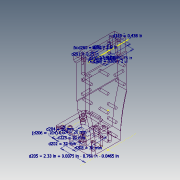
# Autodesk Inventor part: J003055
Saved by Autodesk Inventor 2015 SP1 (Build 190203100, 203)
## iProperties
Created: 2014-12-15
Material: ALUMINUM, 6061-T651
Vendor: HHMI: JFRC - ID&F
Document SubType Name: Modeling
Designer: ARNOLDJ
Density: 2.7 g/cm^3
Mass: 360.292 g
Surface Area: 312.552 cm^2
Volume: 133.442 cm^3
Part Number: J003055
Description: MBS OUTER POSARM
Appearance: Polished Brushed
Project: P-201804
RuleStatus: InUse
AfterDocSave0: file://Part Number Cleaner
LAB/DEPT: SVOBODA (LAB)
REQUESTING SCIENTIST: SOFRONIEW, NICK
SURFACE ROUGHNESS: 63 Ra
DESIGN DEPARTMENT: HHMI: JRC - ID&F
SPECIAL FINISH: ANODIZE PER MIL-A-8625F, TYPE II, CLASS 2 (BLACK)
ALTERED ITEM PART NUMBER: N/A
ALTERED ITEM VENDOR: N/A
ALTERED ITEM DESCRIPTION: N/A
Revision Number: -
Autodesk Inventor part; units mm, degrees
ref_plane "XZ Plane" through (0, 0, 0) normal (0, 1, 0) x (-1, 0, 0)
ref_plane "XY Plane" through (0, 0, 0) normal (0, 0, 1) x (1, 0, 0)
sketch "Sketch1" plane through (0, 0, 0) normal (0, 0, 1) x (1, 0, 0)
  line L0 (0, 106.1009) -> (0, -79.7357) projected
  line L1 (-19.05, 0) -> (3.175, 0) projected
  line L2 (-15.875, -53.1876) -> (-15.875, 79.5528)
  line L3 (0, -53.1876) -> (0, 79.5528)
  line L4 (-15.875, 79.5528) -> (0, 79.5528)
  line L5 (0, -53.1876) -> (-15.875, -53.1876)
  line L6 (-7.9375, 79.5528) -> (-7.9375, -53.1876) construction
  point P0 (0, 0)
  dimension "d5" = 15.875
  dimension "d67" = 0
  dimension "d118" = 53.1876
  dimension "d119" = 79.5528
  constraints: 10 end point, 2 horizontal, 2 midpoint, 1 perpendicular, 1 vertical
  measures "d5" distance between parallel lines of L2 L3
  measures "d67" distance between parallel lines of L0 L3
  measures "d118" distance between parallel lines of L5 L1
  measures "d119" distance between parallel lines of L1 L4
extrude "Extrusion1" add sketch "Sketch1" along normal mid plane 63.5
sketch "Sketch17" plane through (-15.875, -53.1876, 31.75) normal (0, -1, 0) x (1, 0, 0)
  line L0 (0, -9.25) -> (-44.1706, -9.25)
  line L1 (0, 0) -> (0, -63.5) projected
  line L2 (-44.1706, -9.25) -> (-44.1706, -54.25)
  line L3 (-44.1706, -54.25) -> (0, -54.25)
  line L4 (0, -63.5) -> (0, 0)
  line L5 (-55.423, -31.75) -> (27.758, -31.75) projected
  point P0 (15.875, -31.75)
  dimension "d190" = 45
  dimension "d191" = 22.5
  dimension "d384" = 44.1706
  constraints: 8 end point, 4 perpendicular, 2 point on line
  measures "d190" distance of L0.end L2.end
  measures "d191" distance between parallel lines of L5 L0
  measures "d384" distance between parallel lines of L1 L2
extrude "Extrusion9" add sketch "Sketch17" against normal blind 12.7
sketch "Sketch18" plane through (-15.875, -40.4876, 31.75) normal (0, 1, 0) x (1, 0, 0)
  line L0 (-44.1706, 9.25) -> (0, 9.25) projected
  line L1 (-40.3606, 9.25) -> (-14.9606, 9.25)
  line L2 (-14.9606, 9.25) -> (-14.9606, 11.75)
  line L3 (-14.9606, 11.75) -> (-40.3606, 11.75)
  line L4 (-40.3606, 11.75) -> (-40.3606, 9.25)
  line L5 (-44.1706, 54.25) -> (-44.1706, 9.25) projected
  line L6 (0, 0) -> (0, 63.5) projected
  line L7 (0, 54.25) -> (-44.1706, 54.25) projected
  line L8 (-40.3606, 54.25) -> (-14.9606, 54.25)
  line L9 (-14.9606, 54.25) -> (-14.9606, 52.1418)
  line L10 (-14.9606, 52.1418) -> (-40.3606, 52.1418)
  line L11 (-40.3606, 52.1418) -> (-40.3606, 54.25)
  point P0 (15.875, 31.75)
  point P1 (-9.25, 9.25)
  dimension "d215" = 2.5
  dimension "d217" = 3.81
  dimension "d218" = 25.4
  dimension "d258" = 14.9606
  dimension "d385" = 2.1082
  constraints: 16 end point, 4 parallel, 2 horizontal, 2 perpendicular, 2 point on line, 2 vertical alignment
  measures "d215" distance of L1.end L2.end
  measures "d217" distance between parallel lines of L5 L4
  measures "d218" distance of L2.end L3.end
  measures "d258" distance from line of L1.end L6
  measures "d385" distance of L8.end L9.end
extrude "Extrusion10" add sketch "Sketch18" along normal blind 1.524 contours L4 L3 L2 L0 | L7 L9 L10 L11
sketch "Sketch19" plane through (0, -53.1876, -31.75) normal (0, -1, 0) x (1, 0, 0)
  line L0 (-54.862, 47.75) -> (-22.862, 47.75) construction
  line L1 (-22.862, 47.75) -> (-22.862, 15.75) construction
  line L2 (-22.862, 15.75) -> (-54.862, 15.75) construction
  line L3 (-54.862, 15.75) -> (-54.862, 47.75) construction
  line L4 (-72.0547, 31.75) -> (12.0091, 31.75) construction
  line L5 (-38.862, 47.75) -> (-38.862, 15.75) construction
  line L6 (0, 76.2) -> (0, -12.7) construction
  line L7 (-60.0456, 54.25) -> (-60.0456, 9.25) construction
  line L8 (-28.862, 21.75) -> (-48.862, 21.75) construction
  line L9 (-48.862, 21.75) -> (-48.862, 41.75) construction
  line L10 (-48.862, 41.75) -> (-28.862, 41.75) construction
  line L11 (-28.862, 41.75) -> (-28.862, 21.75) construction
  line L12 (-28.862, 21.75) -> (-48.862, 41.75) construction
  line L13 (-48.862, 21.75) -> (-28.862, 41.75) construction
  point P0 (0, 31.75)
  point P1 (-38.862, 31.75)
  dimension "d202" = 32
  dimension "d203" = 32
  dimension "d204" = 16
  dimension "d205" = 38.862
  dimension "d206" = 5.1836
  dimension "d223" = 20
  dimension "d224" = 20
  constraints: 22 end point, 5 midpoint, 4 parallel, 2 horizontal, 2 perpendicular
  measures "d202" distance of L0.start L0.end
  measures "d203" distance of L0.end L1.end
  measures "d204" distance between parallel lines of L4 L0
  measures "d205" distance between parallel lines of L6 L5
  measures "d206" distance between parallel lines of L7 L3
  measures "d223" distance of L9.end L10.end
  measures "d224" distance of L8.end L9.end
hole "Hole8" at (-54.862, -53.1876, 16) at (-22.862, -53.1876, 16) at (-22.862, -53.1876, -16) at (-54.862, -53.1876, -16) direction (0, 1, 0) diameter 3.6068 end through all counterbore diameter 8.255 counterbore depth 9.9314 clearance for "Socket Head Cap Screw" size "M3" standard "Ansi Metric M Profile"
hole "Hole9" at (-48.862, -53.1876, 10) at (-28.862, -53.1876, 10) at (-28.862, -53.1876, -10) at (-48.862, -53.1876, -10) direction (0, 1, 0) diameter 3.175 end through all counterbore diameter 6.35 counterbore depth 10.4394
sketch "Sketch25" plane through (0, 0, 0) normal (0, 0, 1) x (1, 0, 0)
  line L0 (-15.875, 79.5528) -> (0, 79.5528) projected
  line L1 (0, 79.5528) -> (0, -53.1876) projected
  line L2 (0, 79.5528) -> (-5.08, 79.5528)
  line L3 (-5.08, 79.5528) -> (-5.08, 61.3156)
  line L4 (-5.08, 61.3156) -> (0, 61.3156)
  line L5 (0, 61.3156) -> (0, 79.5528)
  point P0 (0, 0)
  dimension "d280" = 5.08
  dimension "d281" = 18.2372
  constraints: 8 end point, 2 parallel, 1 horizontal, 1 perpendicular
  measures "d280" distance of L3.end L4.end
  measures "d281" distance of L2.end L3.end
extrude "Extrusion13" cut sketch "Sketch25" along normal mid plane 76.2
sketch "Sketch26" plane through (0, 0, 0) normal (0, 0, 1) x (1, 0, 0)
  line L0 (-15.875, 79.5528) -> (0, 79.5528) projected
  line L1 (-15.875, -53.1876) -> (-15.875, 79.5528) projected
  line L2 (-15.875, 79.5528) -> (-21.844, 79.5528)
  line L3 (-21.844, 79.5528) -> (-21.844, 70.6628)
  line L4 (-21.844, 70.6628) -> (-15.875, 70.6628)
  line L5 (-15.875, 70.6628) -> (-15.875, 79.5528)
  line L6 (-15.875, 70.6628) -> (-17.145, 70.6628)
  line L7 (-17.145, 70.6628) -> (-17.145, 19.8628)
  line L8 (-17.145, 19.8628) -> (-15.875, 19.8628)
  line L9 (-15.875, 19.8628) -> (-15.875, 70.6628)
  point P0 (0, 0)
  point P1 (-5.08, 79.5528)
  point P2 (-15.875, 56.6928)
  dimension "d284" = 5.969
  dimension "d285" = 8.89
  dimension "d313" = 22.86
  dimension "d317" = 50.8
  dimension "d318" = 1.27
  constraints: 16 end point, 4 parallel, 2 horizontal, 2 perpendicular, 1 point on line
  measures "d284" distance of L3.end L4.end
  measures "d285" distance of L2.end L3.end
  measures "d313" distance from line of L0 point (-15.875, 56.693)
  measures "d317" distance of L6.end L7.end
  measures "d318" distance of L7.end L8.end
extrude "Extrusion14" add sketch "Sketch26" along normal up to surface (63.5 mm away) from surface at -31.75
sketch "Sketch27" plane through (-15.875, -53.1876, 31.75) normal (0, -1, 0) x (1, 0, 0)
  point P0 (15.875, -31.75)
sketch "Sketch28" plane through (-15.875, -53.1876, 31.75) normal (0, -1, 0) x (1, 0, 0)
  line L0 (0, -9.25) -> (-44.1706, -9.25) projected
  line L1 (-44.1706, -9.25) -> (-44.1706, -54.25) construction
  line L2 (-44.1706, -54.25) -> (0, -54.25) projected
  line L3 (0, -54.25) -> (-44.1706, -54.25) projected
  line L4 (-44.1706, -9.25) -> (-21.3106, -9.25)
  line L5 (-21.3106, -9.25) -> (-21.3106, -54.25)
  line L6 (-21.3106, -54.25) -> (-44.1706, -54.25)
  line L7 (-44.1706, -54.25) -> (-44.1706, -9.25)
  point P0 (15.875, -31.75)
  dimension "d302" = 22.86
  constraints: 8 end point, 2 parallel, 1 horizontal, 1 perpendicular, 1 point on line
  measures "d302" distance from line of L5 L0.end
extrude "Extrusion15" cut sketch "Sketch28" against normal blind 6.35
fillet "Fillet10" radius 3.175 2 edges at (-60.0456, -43.6626, 22.5) (-60.0456, -43.6626, -22.5)
sketch "Sketch20" plane through (0, 0, 0) normal (1, 0, 0) x (0, 1, 0)
  line L0 (-53.1876, -31.75) -> (-53.1876, 31.75) projected
  line L1 (-53.1876, -31.75) -> (79.5528, -31.75) projected
  line L2 (-41.7576, 12.7) -> (-3.6576, 12.7) construction
  line L3 (-3.6576, 12.7) -> (-3.6576, -12.7) construction
  line L4 (-3.6576, -12.7) -> (-41.7576, -12.7) construction
  line L5 (-41.7576, -12.7) -> (-41.7576, 12.7) construction
  line L6 (-79.7331, 0) -> (106.0856, 0) construction
  line L7 (21.7424, 25.4) -> (21.7424, -25.4)
  line L8 (21.7424, 25.4) -> (47.1424, 25.4)
  line L9 (47.1424, 25.4) -> (47.1424, -25.4)
  line L10 (47.1424, -25.4) -> (21.7424, -25.4)
  line L11 (21.7424, -25.4) -> (21.7424, 25.4)
  line L12 (26.88, 21.59) -> (43.3324, 21.59)
  line L13 (43.3324, 21.59) -> (43.3324, 3.81)
  line L14 (43.3324, 3.81) -> (26.88, 3.81)
  line L15 (26.88, 3.81) -> (26.88, 21.59)
  line L16 (25.5524, -3.81) -> (43.3324, -3.81)
  line L17 (43.3324, -3.81) -> (43.3324, -21.59)
  line L18 (43.3324, -21.59) -> (25.5524, -21.59)
  line L19 (25.5524, -21.59) -> (25.5524, -3.81)
  point P0 (0, 0)
  point P1 (-53.1876, -23.495)
  point P2 (-53.1876, 23.495)
  point P3 (-44.9326, -31.75)
  point P4 (21.7424, 0)
  point P5 (47.1424, 0)
  point P6 (-22.7076, 12.7)
  point P7 (-22.7076, -12.7)
  point P8 (-22.7076, 0)
  point P9 (-41.7576, 0)
  point P10 (-3.6576, 0)
  dimension "d350" = 25.4
  dimension "d351" = 38.1
  dimension "d352" = 12.7
  dimension "d353" = 11.43
  dimension "d354" = 25.4
  dimension "d355" = 50.8
  dimension "d356" = 25.4
  dimension "d360" = 3.81
  dimension "d361" = 3.81
  dimension "d362" = 3.81
  dimension "d363" = 3.81
  dimension "d364" = 7.62
  dimension "d365" = 3.81
  dimension "d366" = 16.4523
  constraints: 34 end point, 8 coincident, 8 parallel, 6 midpoint, 4 horizontal, 4 perpendicular, 4 point on line, 1 symmetric about line, 1 vertical, 1 other
  measures "d350" distance of L4.end L2.start
  measures "d351" distance of L2.start L2.end
  measures "d352" distance between parallel lines of L6 L2
  measures "d353" distance between parallel lines of L0 L5
  measures "d354" distance between parallel lines of L7 L3
  measures "d355" distance of L7.start L7.end
  measures "d356" distance of L8.start L8.end
  measures "d360" distance between parallel lines of L11 L19
  measures "d361" distance between parallel lines of L9 L13
  measures "d362" distance between parallel lines of L8 L12
  measures "d363" distance between parallel lines of L10 L18
  measures "d364" distance between parallel lines of L14 L16
  measures "d365" distance between parallel lines of L14 L6
  measures "d366" distance of L12.start L12.end
hole "Hole10" at (0, -41.7576, 12.7) at (0, -41.7576, -12.7) at (0, -3.6576, 12.7) at (0, -3.6576, -12.7) at (0, 21.7424, -25.4) at (0, 47.1424, -25.4) at (0, 47.1424, 25.4) at (0, 21.7424, 25.4) at (0, 47.1424, 0) at (0, 21.7424, 0) at (0, -41.7576, 0) at (0, -22.7076, -12.7) at (0, -22.7076, 0) at (0, -22.7076, 12.7) at (0, -3.6576, 0) direction (-1, 0, 0) diameter 3.2512 depth 12.7 tip angle 118
sketch "Sketch21" plane through (-56.8706, -53.1876, 22.5) normal (0, -1, 0) x (1, 0, 0)
  line L0 (-3.175, 0) -> (-3.175, -45) construction
  line L1 (56.8706, 21.95) -> (56.8706, -66.95) construction
  line L2 (-3.175, -41.825) -> (-3.175, -3.175) construction
  line L3 (-3.175, -22.5) -> (56.8706, -22.5) construction
  point P0 (46.7106, -35.2)
  point P1 (46.7106, -9.8)
  point P2 (46.7106, -22.5)
  dimension "d245" = 10.16
  dimension "d370" = 12.7
  dimension "d371" = 12.7
  constraints: 2 end point, 2 vertical alignment, 1 midpoint, 1 perpendicular, 1 point on line
  measures "d245" distance from line of L1 point (46.711, -35.2)
  measures "d370" distance from line of L3 point (46.711, -35.2)
  measures "d371" distance from line of L3 point (46.711, -9.8)
hole "Hole11" at (-10.16, -53.1876, -12.7) at (-10.16, -53.1876, 0) at (-10.16, -53.1876, 12.7) direction (0, 1, 0) diameter 3.2512 depth 12.7 tip angle 118
ref_plane "Work Plane2" through (-38.862, 0, 0) normal (1, 0, 0) x (0, 1, 0)
sketch "Sketch23" plane through (-15.875, 79.5528, 31.75) normal (0, 1, 0) x (1, 0, 0)
  line L0 (4.7625, 0) -> (4.7625, 63.5) construction
  line L1 (15.875, 63.5) -> (15.875, 0) projected
  point P0 (15.875, 31.75)
  point P1 (4.7625, 5.08)
  point P2 (4.7625, 19.05)
  point P3 (4.7625, 44.45)
  point P4 (4.7625, 58.42)
  point P5 (-1.5875, 9.525)
  point P6 (-1.5875, 53.975)
  dimension "d260" = 12.7
  dimension "d261" = 25.4
  dimension "d262" = 26.67
  dimension "d263" = 53.34
  dimension "d289" = 44.45
  dimension "d290" = 22.225
  dimension "d291" = 6.35
  dimension "d319" = 11.1125
  constraints: 4 point on line, 2 end point, 1 vertical alignment
  measures "d260" vertical distance of point (15.875, 31.75) point (4.763, 19.05)
  measures "d261" distance of point (4.763, 44.45) point (4.763, 19.05)
  measures "d262" vertical distance of point (15.875, 31.75) point (4.763, 5.08)
  measures "d263" distance of point (4.763, 5.08) point (4.763, 58.42)
  measures "d289" distance of point (-1.587, 53.975) point (-1.587, 9.525)
  measures "d290" vertical distance of point (15.875, 31.75) point (-1.587, 9.525)
  measures "d291" distance from line of point (-1.587, 9.525) L0
  measures "d319" distance between parallel lines of L0 L1
hole "Hole12" at (-11.1125, 79.5528, 26.67) at (-11.1125, 79.5528, -26.67) direction (0, -1, 0) diameter 4.7498 depth 22.86 tip angle 118 counterbore diameter 4.7879 counterbore depth 5.08
hole "Hole13" at (-17.4625, 79.5528, 22.225) at (-17.4625, 79.5528, -22.225) at (-11.1125, 79.5528, 12.7) at (-11.1125, 79.5528, -12.7) direction (0, -1, 0) diameter 3.2512 depth 14.605 tip angle 118
sketch "Sketch37" plane through (0, -53.1876, 31.75) normal (1, 0, 0) x (0, 0, -1)
  point P0 (31.75, 53.1876)
sketch "Sketch24" plane through (0, 0, 0) normal (1, 0, 0) x (0, 1, 0)
  line L0 (-53.1876, -22.5) -> (-40.4876, -22.5)
  line L1 (9.6224, -31.75) -> (-53.1876, -31.75)
  line L2 (-53.1876, -31.75) -> (-53.1876, -22.5)
  line L3 (-40.4876, -22.5) -> (-40.4876, -31.75) construction
  line L4 (19.8628, -31.75) -> (-53.1876, -31.75) construction
  line L5 (0, 73.0782) -> (0, -216.2191) projected
  line L6 (-79.7357, 0) -> (106.1009, 0) projected
  line L7 (100.3486, 0) -> (-143.1864, 0) construction
  arc A0 (9.6224, -31.75) -> (-40.4876, -22.5) centre (-52.0278, -225.372) ccw
  point P0 (0, 0)
  point P1 (-53.1876, -31.75)
  point P2 (19.8628, 31.75)
  dimension "d375" = 62.81
  dimension "d381" = 12.7
  dimension "d382" = 203.2
  dimension "d383" = 9.25
  constraints: 10 end point, 3 point on line, 2 point on circle, 1 centre point, 1 coincident, 1 horizontal, 1 parallel, 1 perpendicular
  measures "d375" distance of L1.start L1.end
  measures "d381" distance of L0.start L0.end
  measures "d382" radius of A0
  measures "d383" distance of L1.end L0.start
extrude "Extrusion12" cut sketch "Sketch24" against normal up to next
mirror "Mirror1" about plane through (0, 0, 0) normal (0, 0, 1) of "Extrusion12"
chamfer "Chamfer6" distance 1.905 angle 45 1 edges at (-21.844, 70.6628, 0)
chamfer "Chamfer7" distance 3.175 angle 45 1 edges at (-37.1856, -53.1876, 0)
chamfer "Chamfer10" distance 3.175 angle 45 1 edges at (0, -53.1876, 0)
chamfer "Chamfer11" distance 3.175 angle 45 7 edges at (0, -45.2501, -22.5) (0, 35.469, -31.75) (0, 61.3156, 0) (0, 35.469, 31.75) (0, -45.2501, 22.5) (0, -15.1415, -25.548) (0, -15.1415, 25.548)
sketch "Sketch39" plane through (0, 0, -31.75) normal (0, 0, -1) x (-1, 0, 0)
  line L0 (17.145, 19.8628) -> (17.145, 70.6628) projected
  line L1 (15.875, -40.4876) -> (30.8356, -40.4876) projected
  line L2 (8.5725, 51.9684) -> (8.5725, 32.9184) construction
  line L3 (0, 58.1406) -> (0, 10.1137) construction
  circle A0 centre (8.5725, 32.9184) radius 2.0003 construction
  circle A1 centre (8.5725, 51.9684) radius 2.0003 construction
  line L4 (3.175, 9.6224) -> (3.175, 61.3156) construction
  line L5 (3.175, 9.6224) -> (15.875, 9.6224) construction
  line L6 (15.875, 19.8628) -> (15.875, 9.6224) construction
  line L7 (15.875, 19.8628) -> (17.145, 19.8628) construction
  line L8 (17.145, 19.8628) -> (17.145, 70.6628) construction
  line L9 (17.145, 70.6628) -> (19.939, 70.6628) construction
  line L10 (21.844, 72.5678) -> (19.939, 70.6628) construction
  line L11 (21.844, 72.5678) -> (21.844, 79.5528) construction
  line L12 (21.844, 79.5528) -> (5.08, 79.5528) construction
  line L13 (5.08, 79.5528) -> (5.08, 61.3156) construction
  line L14 (5.08, 61.3156) -> (3.175, 61.3156) construction
  point P0 (0, 0)
  dimension "d391" = 8.5725
  dimension "d392" = 17.145
  dimension "d394" = 4.0005
  dimension "d395" = 4.0005
  dimension "d403" = 92.456
  dimension "d404" = 19.05
  dimension "d405" = 27.5844
  constraints: 4 coincident, 2 centre point, 2 end point, 1 vertical
  measures "d391" distance between parallel lines of L2 L0
  measures "d392" distance between parallel lines of L3 L0
  measures "d394" diameter of A0
  measures "d395" diameter of A1
  measures "d403" distance from line of L1 L2.start
  measures "d404" distance of L2.start L2.end
  measures "d405" distance from line of L12 point (8.572, 51.968)
hole "Hole14" at (-8.5725, 32.9184, -31.75) at (-8.5725, 51.9684, -31.75) direction (0, 0, 1) diameter 3.2512 depth 12.7 tip angle 118
sketch "Sketch40" plane through (0, 0, 31.75) normal (0, 0, 1) x (1, 0, 0)
  circle A0 centre (-8.5725, 51.9684) radius 1.6256 projected
  circle A1 centre (-8.5725, 32.9184) radius 1.6256 projected
  point P0 (0, 0)
  constraints: 2 coincident
hole "Hole15" at (-8.5725, 51.9684, 31.75) at (-8.5725, 32.9184, 31.75) direction (0, 0, -1) diameter 3.2512 depth 12.7 tip angle 118
body "Solid1"
